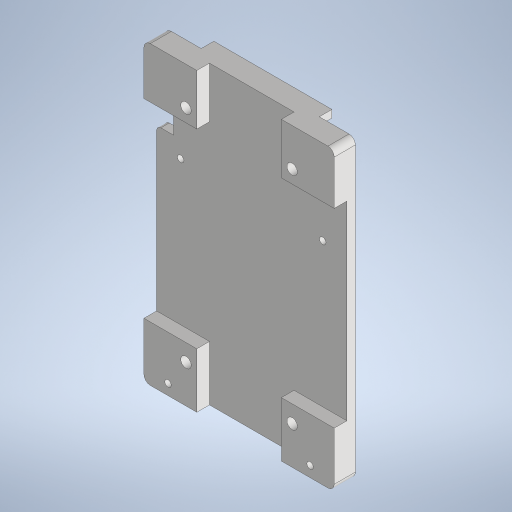
# Autodesk Inventor part: 와이파이 모듈 커버
Saved by Autodesk Inventor 2023 (Build 270158000, 158)
## iProperties
Created: 2022-06-24
Part Number: 와이파이 모듈 커버
Material: 일반
Document SubType Name: Modeling
Designer: user
Density: 1 g/cm^3
Appearance: 기본값
Author: user
Autodesk Inventor part; units mm, degrees
ref_plane "YZ Plane" through (0, 0, 0) normal (1, 0, 0) x (0, 1, 0)
ref_plane "XZ Plane" through (0, 0, 0) normal (0, 1, 0) x (-1, 0, 0)
ref_plane "XY Plane" through (0, 0, 0) normal (0, 0, 1) x (1, 0, 0)
sketch "스케치1" plane through (0, 0, 0) normal (0, 0, 1) x (1, 0, 0)
  line L0 (-21, 35) -> (21, 35)
  line L1 (22.5, 33.5) -> (22.5, -33.5)
  line L2 (21, -35) -> (-21, -35)
  line L3 (-22.5, -33.5) -> (-22.5, 33.5)
  line L4 (-22.5, 35) -> (22.5, -35) construction
  line L5 (22.5, 35) -> (-22.5, -35) construction
  circle A0 centre (-12.55, 26.05) radius 1.25
  line L6 (0, 0) -> (0, 21.4248) construction
  line L7 (0, 0) -> (10.8427, 0) construction
  circle A1 centre (12.55, 26.05) radius 1.25
  circle A2 centre (-12.55, -26.05) radius 1.25
  circle A3 centre (12.55, -26.05) radius 1.25
  arc A4 (-21, 35) -> (-22.5, 33.5) centre (-21, 33.5) ccw
  arc A5 (22.5, 33.5) -> (21, 35) centre (21, 33.5) ccw
  arc A6 (21, -35) -> (22.5, -33.5) centre (21, -33.5) ccw
  arc A7 (-22.5, -33.5) -> (-21, -35) centre (-21, -33.5) ccw
  line L8 (-22.5, 23) -> (22.5, 23)
  line L9 (-22.5, -22) -> (22.5, -22)
  line L10 (-10, 3.7) -> (10, 3.7)
  line L11 (10, 3.7) -> (10, 23)
  line L12 (10, 23) -> (-10, 23)
  line L13 (-10, 23) -> (-10, 3.7)
  line L14 (-10, 3.7) -> (10, 23) construction
  line L15 (10, 3.7) -> (-10, 23) construction
  line L16 (10, -3.7) -> (10, -23)
  line L17 (-10, -23) -> (-10, -3.7)
  line L18 (10, 23) -> (10, 35)
  line L19 (-10, 23) -> (-10, 35)
  line L20 (-10, -23) -> (-10, -35)
  line L21 (10, -23) -> (10, -35)
  point P0 (0, 13.35)
  point P1 (10, 13.35)
  point P2 (-10, -28.8)
  point P3 (-10, -22)
  point P4 (10, -22)
  point P5 (10, -28.8)
  point P6 (-10, 23)
  point P7 (-10, 28.8)
  point P8 (10, 28.8)
  dimension "d0" = 45
  dimension "d1" = 70
  dimension "d2" = 25.1
  dimension "d3" = 52.1
  dimension "d4" = 2.5
  dimension "d5" = 1.5
  dimension "d6" = 12
  dimension "d7" = 13
  dimension "d8" = 20
  constraints: 44 end point, 17 point on line, 8 centre point, 8 perpendicular, 8 point on circle, 8 tangent, 7 symmetric about line, 5 midpoint, 4 parallel, 3 equal radius, 3 horizontal, 1 vertical, 1 vertical alignment, 3 other
  measures "d0" distance of L4.end L5.end
  measures "d1" distance of L5.start L4.end
  measures "d2" distance of A1.centre A0.centre
  measures "d3" distance of A2.centre A0.centre
  measures "d4" diameter of A0
  measures "d5" radius of A4
  measures "d6" distance between parallel lines of L0 L8
  measures "d7" distance between parallel lines of L2 L9
  measures "d8" distance from line of point (10, 13.35) L13
extrude "돌출1" add sketch "스케치1" along normal blind 3 contours L0 L19 L8 L3 A4 | L0 A5 L1 L8 L18 | L9 L17 L20 L2 A7 L3 | L1 A6 L2 L21 L16 L9
extrude "돌출2" add sketch "스케치1" against normal blind 2
sketch "스케치3" plane through (0, 0, -2) normal (0, 0, -1) x (-1, 0, 0)
  line L0 (16.8, 12) -> (-16.8, 12) construction
  line L1 (-16.8, 12) -> (-16.8, -32.5) construction
  line L2 (-16.8, -32.5) -> (16.8, -32.5) construction
  line L3 (16.8, -32.5) -> (16.8, 12) construction
  line L4 (16.8, 12) -> (-16.8, -32.5) construction
  line L5 (-16.8, 12) -> (16.8, -32.5) construction
  circle A0 centre (16.8, 12) radius 2.5
  circle A1 centre (16.8, -32.5) radius 2.5
  circle A2 centre (-16.8, 12) radius 2.5
  circle A3 centre (-16.8, -32.5) radius 2.5
  line L6 (-21, -35) -> (21, -35) projected
  point P0 (0, 0)
  point P1 (0, -10.25)
  point P2 (0, 12)
  dimension "d13" = 44.5
  dimension "d14" = 33.6
  dimension "d34" = 5
  dimension "d35" = 5
  dimension "d36" = 5
  dimension "d37" = 5
  constraints: 12 end point, 4 centre point, 4 coincident, 3 midpoint, 2 parallel, 1 horizontal, 1 perpendicular, 1 tangent, 1 vertical alignment
  measures "d13" distance of L2.end L0.start
  measures "d14" distance of L1.end L2.end
  measures "d34" diameter of A0
  measures "d35" diameter of A1
  measures "d36" diameter of A2
  measures "d37" diameter of A3
sketch "스케치4" plane through (0, 0, -2) normal (0, 0, -1) x (-1, 0, 0)
  circle A0 centre (12.55, -26.05) radius 1.25 projected
  circle A1 centre (12.55, -26.05) radius 1.75
  circle A2 centre (-12.55, -26.05) radius 1.25 projected
  circle A3 centre (-12.55, -26.05) radius 1.75
  circle A4 centre (12.55, 26.05) radius 1.25 projected
  circle A5 centre (12.55, 26.05) radius 1.75
  circle A6 centre (-12.55, 26.05) radius 1.75
  point P0 (0, 0)
  dimension "d22" = 3.5
  dimension "d23" = 3.5
  dimension "d24" = 3.5
  dimension "d25" = 3.5
  constraints: 4 centre point, 3 coincident
  measures "d22" diameter of A1
  measures "d23" diameter of A3
  measures "d24" diameter of A5
  measures "d25" diameter of A6
extrude "돌출3" cut sketch "스케치4" against normal blind 2 contours A0 | A1 | A2 | A3 | A4 | A5 | A6
sketch "스케치5" plane through (0, 0, -2) normal (0, 0, -1) x (-1, 0, 0)
  line L0 (13.97, 15.75) -> (-13.97, 15.75)
  line L1 (-13.97, 15.75) -> (-13.97, 33.25)
  line L2 (-13.97, 33.25) -> (13.97, 33.25)
  line L3 (13.97, 33.25) -> (13.97, 15.75)
  line L4 (13.97, 15.75) -> (-13.97, 33.25) construction
  line L5 (-13.97, 15.75) -> (13.97, 33.25) construction
  line L6 (13.97, 14) -> (-13.97, 14)
  line L7 (-13.97, 14) -> (-13.97, 35)
  line L8 (-13.97, 35) -> (13.97, 35)
  line L9 (13.97, 35) -> (13.97, 14)
  line L10 (13.97, 14) -> (-13.97, 35) construction
  line L11 (-13.97, 14) -> (13.97, 35) construction
  line L12 (21, 35) -> (-21, 35) projected
  point P0 (0, 0)
  point P1 (0, 24.5)
  point P2 (-13.97, 33.25)
  point P3 (13.97, 33.25)
  point P4 (13.97, 15.75)
  point P5 (-13.97, 15.75)
  point P6 (0, 35)
  dimension "d28" = 27.94
  dimension "d29" = 17.5
  dimension "d30" = 21
  constraints: 24 end point, 6 midpoint, 4 parallel, 2 horizontal, 2 perpendicular, 1 vertical alignment
  measures "d28" distance of L0.start L0.end
  measures "d29" distance of L0.end L1.end
  measures "d30" distance between parallel lines of L8 L6
extrude "돌출4" add sketch "스케치5" along normal blind 3 contours L9 L6 L7 L0 | L2 L7 L8 L9
extrude "돌출6" add sketch "스케치3" along normal blind 3
sketch "스케치7" plane through (-16.8, 12, -5) normal (0, 0, -1) x (-1, 0, 0)
  circle A0 centre (0, 0) radius 2.5 projected
  circle A1 centre (0, -44.5) radius 2.5 projected
  circle A2 centre (-33.6, 0) radius 2.5 projected
  circle A3 centre (-33.6, -44.5) radius 2.5 projected
  point P0 (-16.8, -12)
hole "구멍3" at (-16.8, 12, -5) at (-16.8, -32.5, -5) at (16.8, -32.5, -5) at (16.8, 12, -5) direction (0, 0, 1) diameter 1.567 end through all countersink diameter 3 countersink angle 90 thread size "M2x0.4" class "6H" standard "ISO Metric profile"
sketch "스케치9" plane through (0, 0, 0) normal (0, 0, 1) x (1, 0, 0)
  line L0 (-22.5, 33.5) -> (-22.5, 23) projected
  line L1 (-22.5, 23) -> (-18.5, 23)
  line L2 (-18.5, 23) -> (-18.5, 16)
  line L3 (-18.5, 16) -> (-22.5, 16)
  line L4 (-22.5, 16) -> (-22.5, 23)
  point P0 (0, 0)
  dimension "d58" = 4
  dimension "d59" = 7
  constraints: 8 end point, 2 parallel, 1 horizontal, 1 perpendicular
  measures "d58" distance of L2.end L3.end
  measures "d59" distance of L1.end L2.end
extrude "돌출7" cut sketch "스케치9" against normal blind 2
fillet "모깎기1" radius 1 1 edges at (-22.5, 16, -1)
